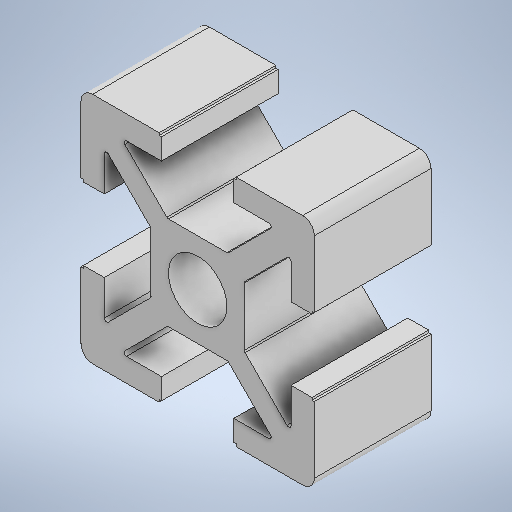
# Autodesk Inventor part: profile_20x20_0001_0001
Saved by Autodesk Inventor 2025.2 (Build 292293000, 293)
## iProperties
Created: 2025-03-25
Part Number: profile_20x20_0001_0001
Material: Generic
Document SubType Name: Modeling
Designer: kenne
Density: 1 g/cm^3
Appearance: Default
Author: kenne
Autodesk Inventor part; units mm, degrees
ref_plane "YZ Plane" through (0, 0, 0) normal (1, 0, 0) x (0, 1, 0)
ref_plane "XZ Plane" through (0, 0, 0) normal (0, 1, 0) x (-1, 0, 0)
ref_plane "XY Plane" through (0, 0, 0) normal (0, 0, 1) x (1, 0, 0)
sketch "Sketch1" plane through (0, 0, 0) normal (0, 0, 1) x (1, 0, 0)
  line L0 (-10, 10) -> (10, 10) construction
  circle A0 centre (0, 0) radius 2.5 construction
  line L1 (0, 0) -> (-10, 10) construction
  line L2 (-4, 4) -> (4, 4) construction
  line L3 (4, 4) -> (4, -4) construction
  line L4 (4, -4) -> (-4, -4) construction
  line L5 (-4, -4) -> (-4, 4) construction
  line L6 (-4, 4) -> (4, -4) construction
  line L7 (4, 4) -> (-4, -4) construction
  line L8 (-6.5858, 8) -> (-2.5858, 4) construction
  line L9 (-3.1, 11.2929) -> (3.1, 11.2929) construction
  line L10 (-6.5858, 8) -> (-3.1, 8) construction
  line L11 (-3.1, 8) -> (-3.1, 10) construction
  line L12 (-3.1, 10) -> (-10, 10) construction
  line L13 (-10, 10) -> (-10, 3.1) construction
  line L14 (-10, 3.1) -> (-8, 3.1) construction
  line L15 (-8, 3.1) -> (-8, 6.5858) construction
  line L16 (-8, 6.5858) -> (-4, 2.5858) construction
  arc A1 (-6.1029, 8) -> (-6.2444, 7.6586) centre (-6.1029, 7.8) ccw
  line L17 (-6.1029, 8) -> (-3.1, 8)
  arc A2 (-7.6586, 6.2444) -> (-8, 6.1029) centre (-7.8, 6.1029) ccw
  line L18 (-7.6586, 6.2444) -> (-4, 2.5858) construction
  line L19 (-8, 6.1029) -> (-8, 3.1)
  arc A3 (-2.6444, 4.0586) -> (-2.5029, 4) centre (-2.5029, 4.2) ccw
  line L20 (-6.2444, 7.6586) -> (-2.6444, 4.0586)
  line L21 (-2.5858, 4) -> (0, 4)
  arc A4 (-4, 2.5029) -> (-4.0586, 2.6444) centre (-4.2, 2.5029) ccw
  line L22 (-7.6586, 6.2444) -> (-4.0586, 2.6444)
  line L23 (-4, 2.5029) -> (-4, 0)
  arc A5 (0, 2.5) -> (-2.5, 0) centre (0, 0) ccw
  line L24 (-10, 3.1) -> (-10, 3.3) construction
  line L25 (-10, 3.3) -> (-9.8, 3.3)
  line L26 (-9.8, 3.3) -> (-9.8, 3.1)
  line L27 (-9.8, 3.1) -> (-10, 3.1) construction
  line L28 (-9.8, 3.1) -> (-8, 3.1)
  arc A6 (-9, 10) -> (-10, 9) centre (-9, 9) ccw
  line L29 (-10, 9) -> (-10, 3.3)
  line L30 (-3.1, 10) -> (-3.3, 10) construction
  line L31 (-3.3, 10) -> (-3.3, 9.8)
  line L32 (-3.3, 9.8) -> (-3.1, 9.8)
  line L33 (-3.1, 9.8) -> (-3.1, 10) construction
  line L34 (-3.1, 9.8) -> (-3.1, 8)
  line L35 (-9, 10) -> (-3.3, 10)
  line L36 (0, 4) -> (0, 2.5)
  line L37 (-4.0586, 0) -> (-2.5, 0)
  line L38 (-4, 0) -> (-2.5, 0)
  point P0 (0, 10)
  point P1 (0, 11.2929)
  dimension "d0" = 20
  dimension "d1" = 10
  dimension "d2" = 5
  dimension "d3" = 6
  dimension "d4" = 2
  dimension "d5" = 1
  dimension "d6" = 6.2
  dimension "d7" = 1.2929
  dimension "d9" = 2
  dimension "d10" = 3.1
  dimension "d11" = 0.2
  dimension "d12" = 0.2
  dimension "d13" = 0.2
  dimension "d14" = 0.2
  dimension "d15" = 0.2
  dimension "d16" = 1
  dimension "d17" = 0.2
  constraints: 78 end point, 14 point on circle, 13 point on line, 10 tangent, 8 horizontal, 7 centre point, 7 collinear, 6 midpoint, 6 parallel, 5 equal length, 5 vertical, 4 perpendicular, 3 vertical alignment, 1 coincident, 1 horizontal alignment
  measures "d0" distance of L0.start L0.end
  measures "d1" horizontal distance of point (0, 0) L0.start
  measures "d2" diameter of A0
  measures "d3" distance between parallel lines of L0 L2
  measures "d4" distance from line of L0 L8.start
  measures "d5" distance between parallel lines of L1 L8
  measures "d6" distance of L9.start L9.end
  measures "d7" distance between parallel lines of L0 L9
  measures "d9" distance of L13.end L14.end
  measures "d10" distance from line of point (0, 0) L14
  measures "d11" radius of A1
  measures "d12" radius of A2
  measures "d13" radius of A3
  measures "d14" radius of A4
  measures "d15" distance of L25.end L26.end
  measures "d16" radius of A6
  measures "d17" distance of L30.end L31.end
extrude "Extrusion1" add sketch "Sketch1" against normal blind 10
mirror "Mirror1" about plane through (0, 0, 0) normal (1, 0, 0) of "Extrusion1"
mirror "Mirror2" about plane through (0, 0, 0) normal (0, 1, 0) of "Extrusion1", "Mirror1"
equation "\"d1\" = 0.5 * d0"
body "Solid1"
